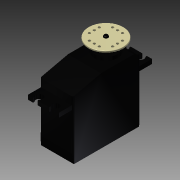
# Autodesk Inventor part: 14-0002
Saved by Autodesk Inventor 2015 SP1 (Build 190203100, 203)
## iProperties
Category: Servo Kit
Company: Autodesk Inc.
Created: 2014-12-02
Part Number: 14-0002
Material: Polystyrene, High Impact
Document SubType Name: Modeling
Designer: Matrix
Density: 1.022 g/cm^3
Appearance: Smooth - Black
Catalog Web Link: http://matrixrobotics.com/
Vendor: Matrix
Author: Autodesk Inc.
Autodesk Inventor part; units mm, degrees
note: some values were not read from the file. Chosen so that the rebuilt part matches the saved one: direction of "Hole2".
ref_plane "YZ Plane" through (0, 0, 0) normal (1, 0, 0) x (0, 1, 0)
sketch "Sketch1" plane through (0, 0, 0) normal (0, 1, 0) x (-1, 0, 0)
  line L0 (0, 0) -> (0, -101.0529) construction
  line L1 (0, -101.0529) -> (-71.6103, -101.0529) construction
  line L2 (-71.6103, -101.0529) -> (-71.6103, 0) construction
  line L3 (-71.6103, 0) -> (0, 0) construction
  line L4 (-62.3914, -23.3491) -> (-62.3914, -64.0491)
  line L5 (-56.738, -24.371) -> (-56.738, -64.0491)
  line L6 (-56.738, -64.0491) -> (-51.4651, -64.4447)
  line L7 (-51.4651, -64.4447) -> (-20.2623, -64.4447)
  line L8 (-20.2623, -64.4447) -> (-17.338, -60.7674)
  line L9 (-17.338, -60.7674) -> (-17.338, -40.9091)
  line L10 (-17.338, -40.9091) -> (-21.2833, -23.7447)
  line L11 (-21.2833, -23.7447) -> (-51.4651, -23.7447)
  line L12 (-51.4651, -23.7447) -> (-56.738, -24.371)
  dimension "d3" = 40.7
  dimension "d6" = 40.7
  dimension "d7" = 39.4
  constraints: 18 end point, 3 vertical, 2 parallel, 1 perpendicular, 1 vertical alignment, 2 other
  measures "d3" distance of L4.start L4.end
  measures "d6" distance between parallel lines of L7 L11
  measures "d7" distance between parallel lines of L9 L5
extrude "Extrusion1" add sketch "Sketch1" against normal blind 20
ref_plane "Work Plane1" through (21.2833, -10, -23.7447) normal (0, 1, 0) x (1, 0, 0)
sketch "Sketch2" plane through (21.2833, -10, -23.7447) normal (0, 1, 0) x (1, 0, 0)
  line L0 (30.1818, 0) -> (0, 0) projected
  line L1 (7.1555, 0) -> (7.1555, -7.8053)
  line L2 (7.1555, -7.8053) -> (4.5593, -7.8053)
  line L3 (4.5593, -7.8053) -> (4.5593, 0)
  point P0 (-21.2833, -23.7447)
  constraints: 6 end point, 2 perpendicular, 2 point on line, 1 vertical
extrude "Extrusion2" add sketch "Sketch2" along normal mid plane 18.8
sketch "Sketch3" plane through (25.8426, -19.4, -15.9394) normal (-1, 0, 0) x (0, 0, 1)
  line L0 (-22.449, -14.3939) -> (-126.4878, -14.3939) construction
  line L1 (-126.4878, -14.3939) -> (-126.4878, 39.9402) construction
  line L2 (-126.4878, 39.9402) -> (-22.449, 39.9402) construction
  line L3 (-22.449, 39.9402) -> (-22.449, -14.3939) construction
  line L4 (0, 0) -> (-7.8053, 0) projected
  line L5 (-6.9631, 10) -> (-2.9631, 10)
  arc A0 (-2.9631, 8.8) -> (-2.9631, 10) centre (-2.9631, 9.4) ccw
  line L6 (-2.9631, 8.8) -> (-6.9631, 8.8)
  line L7 (-7.0833, 0) -> (-0.9, 0)
  arc A1 (-0.9, 0) -> (0, 0.9) centre (-0.9, 0.9) ccw
  line L8 (0, 0.9) -> (0, 3.15)
  line L9 (0, 3.15) -> (-0.7914, 3.15)
  arc A2 (-2.4, 2.4) -> (-0.7914, 3.15) centre (-2.4, 4.5) ccw
  arc A3 (-2.4, 6.6) -> (-2.4, 2.4) centre (-2.4, 4.5) ccw
  arc A4 (-0.7914, 5.85) -> (-2.4, 6.6) centre (-2.4, 4.5) ccw
  line L10 (-0.7914, 5.85) -> (0, 5.85)
  line L11 (0, 5.85) -> (0, 12.95)
  line L12 (0, 12.95) -> (-0.7914, 12.95)
  arc A5 (-2.4, 12.2) -> (-0.7914, 12.95) centre (-2.4, 14.3) ccw
  arc A6 (-2.4, 16.4) -> (-2.4, 12.2) centre (-2.4, 14.3) ccw
  arc A7 (-0.7914, 15.65) -> (-2.4, 16.4) centre (-2.4, 14.3) ccw
  line L13 (-0.7914, 15.65) -> (0, 15.65)
  line L14 (0, 15.65) -> (0, 17.9)
  arc A8 (0, 17.9) -> (-0.9, 18.8) centre (-0.9, 17.9) ccw
  line L15 (-0.9, 18.8) -> (-7.0202, 18.8)
  line L16 (-7.8053, 18.8) -> (0, 18.8) projected
  line L17 (-154.9732, 9.4) -> (44.4248, 9.4) projected
  line L18 (0, 5.85) -> (0, 3.15)
  line L19 (0, 15.65) -> (0, 12.95)
  point P0 (15.9394, 19.4)
  point P1 (-3.3667, 13.7468)
  dimension "d60" = 9.8
  dimension "d63" = 4.9
  dimension "d64" = 1.2
  dimension "d65" = 0.6
  constraints: 26 end point, 18 point on circle, 9 centre point, 2 tangent, 2 vertical, 1 collinear, 2 other
  measures "d60" distance of A2.centre A5.centre
  measures "d63" vertical distance of A0.centre A2.centre
  measures "d64" distance between parallel lines of L5 L6
  measures "d65" distance between parallel lines of L17 L6
extrude "Extrusion3" cut sketch "Sketch3" against normal blind 18
sketch "Sketch4" plane through (0, 0, 0) normal (0, 1, 0) x (1, 0, 0)
  point P0 (0, 0)
fillet "Fillet3" radius 1 4 edges at (36.3742, 0, -23.7447) (36.3742, -20, -23.7447) (35.8637, 0, -64.4447) (35.8637, -20, -64.4447)
sketch "Sketch5" plane through (17.338, 0, -60.7674) normal (-1, 0, 0) x (0, 0, 1)
  line L0 (-16.5663, -10) -> (73.6563, -10) projected
  circle A0 centre (7, -10) radius 7
  line L1 (0, 0) -> (0, -20) projected
  point P0 (60.7674, 0)
  dimension "d68" = 14
  constraints: 1 centre point, 1 point on line, 1 tangent
  measures "d68" diameter of A0
extrude "Extrusion4" add sketch "Sketch5" along normal blind 2
sketch "Sketch6" plane through (15.338, -10, -53.7674) normal (-1, 0, 0) x (0, 0, 1)
  circle A0 centre (0, 0) radius 5
  point P0 (53.7674, 10)
  dimension "d71" = 10
  constraints: 1 centre point
  measures "d71" diameter of A0
extrude "Extrusion5" add sketch "Sketch6" along normal blind 1
ref_plane "Work Plane2" through (8.738, 0, -24.371) normal (1, 0, 0) x (0, 0, -1)
sketch "Sketch7" plane through (8.738, 0, -24.371) normal (1, 0, 0) x (0, 0, -1)
  circle A0 centre (29.3964, -10) radius 5 projected
  circle A1 centre (29.3964, -10) radius 1.25
  point P0 (-24.371, 0)
  dimension "d75" = 2.5
  constraints: 1 centre point, 1 coincident
  measures "d75" diameter of A1
extrude "Extrusion6" add sketch "Sketch7" along normal up to surface (5.6 mm away) contours A1
fillet "Fillet1" radius 0.5 1 edges at (8.738, -10, -52.5174)
ref_plane "Work Plane3" through (21.2833, 0, -44.0947) normal (0, 0, 1) x (1, 0, 0)
mirror "Mirror1" about plane through (21.2833, 0, -44.0947) normal (0, 0, 1) of "Extrusion3", "Extrusion2"
ref_plane "Work Plane4" through (9.738, 0, -24.371) normal (1, 0, 0) x (0, 0, -1)
sketch "Sketch8" plane through (9.738, 0, -24.371) normal (1, 0, 0) x (0, 0, -1)
  circle A0 centre (29.3964, -10) radius 1.25 projected
  circle A1 centre (29.3964, -10) radius 5 projected
  circle A2 centre (29.3964, -10) radius 10.5
  point P0 (-24.371, 0)
  dimension "d80" = 21
  constraints: 1 centre point, 1 coincident
  measures "d80" diameter of A2
extrude "Extrusion7" add sketch "Sketch8" along normal blind 1 contours A1 | A2
fillet "Fillet2" radius 0.2 2 edges at (9.738, -10, -43.2674) (10.738, -10, -43.2674)
sketch "Sketch9" plane through (9.738, -10, -53.7674) normal (-1, 0, 0) x (0, 0, 1)
  circle A0 centre (0, 0) radius 1.25 projected
  point P0 (53.7674, 10)
  point P1 (0, -7)
  point P2 (3, -7)
  point P3 (-3, -7)
  dimension "d84" = 7
  dimension "d85" = 3
  dimension "d86" = 3
  constraints: 2 horizontal alignment, 1 vertical alignment
  measures "d84" distance of point (0, -7) A0.centre
  measures "d85" distance of point (3, -7) point (0, -7)
  measures "d86" distance of point (-3, -7) point (0, -7)
hole "Hole2" at (9.738, -17, -53.7674) at (9.738, -17, -50.7674) at (9.738, -17, -56.7674) direction (1, 0, 0) diameter 1.5 end up to surface
pattern_circular "Circular Pattern1" count 4 over 360 about axis through (9.738, -10, -53.7674) along (1, 0, 0) of "Hole2"
equation "\"d86\" = d85"
body "Solid1"
